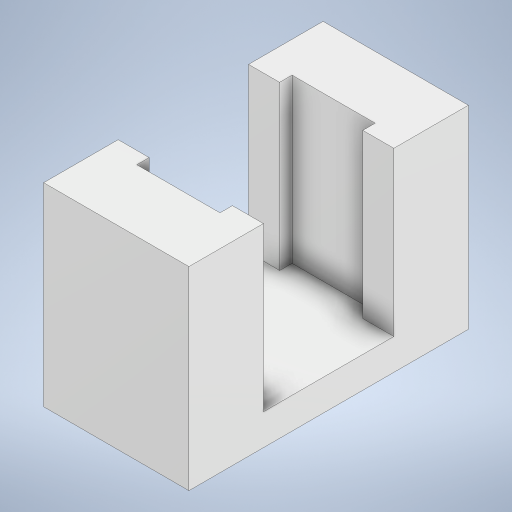
# Autodesk Inventor part: LatchSingleFit
Saved by Autodesk Inventor 2024 (Build 280153000, 153)
## iProperties
Created: 2023-10-31
Part Number: LatchSingleFit
Material: PC/ABS Plastic
Document SubType Name: Modeling
Designer: gcter
Density: 1.1 g/cm^3
Appearance: Smooth - White
Author: gcter
Autodesk Inventor part; units mm, degrees
ref_plane "YZ Plane" through (0, 0, 0) normal (1, 0, 0) x (0, 1, 0)
ref_plane "XZ Plane" through (0, 0, 0) normal (0, 1, 0) x (-1, 0, 0)
ref_plane "XY Plane" through (0, 0, 0) normal (0, 0, 1) x (1, 0, 0)
sketch "Sketch5" plane through (0, 0, 0) normal (0, 1, 0) x (-1, 0, 0)
  line L0 (0, 0) -> (-6.604, 0) construction
  line L1 (-6.604, 0) -> (-6.604, -12.7) construction
  line L2 (-6.604, -12.7) -> (0, -12.7) construction
  line L3 (0, -12.7) -> (0, 0) construction
  line L4 (2.6416, -15.24) -> (-9.2456, -15.24)
  line L5 (-9.2456, -15.24) -> (-9.2456, 2.54)
  line L6 (-9.2456, 2.54) -> (2.6416, 2.54)
  line L7 (2.6416, 2.54) -> (2.6416, -15.24)
  dimension "d22" = 6.604
  dimension "d23" = 12.7
  dimension "d24" = 2.6416
  dimension "d25" = 2.6416
  dimension "d26" = 2.54
  dimension "d27" = 2.54
  constraints: 16 end point, 4 parallel, 2 horizontal, 2 perpendicular
  measures "d22" distance between parallel lines of L1 L3
  measures "d23" distance between parallel lines of L0 L2
  measures "d24" distance between parallel lines of L5 L1
  measures "d25" distance between parallel lines of L3 L7
  measures "d26" distance between parallel lines of L6 L0
  measures "d27" distance between parallel lines of L2 L4
extrude "Extrusion3" add sketch "Sketch5" along normal blind 2.54
sketch "Sketch6" plane through (0, 2.54, 0) normal (0, 1, 0) x (1, 0, 0)
  line L0 (-2.6416, -2.54) -> (9.2456, -2.54)
  line L1 (9.2456, -2.54) -> (9.2456, 0)
  line L2 (6.7056, 0) -> (-0.1016, 0)
  line L3 (-2.6416, -0.508) -> (-2.6416, -2.54)
  line L4 (-2.6416, 15.24) -> (-2.6416, -2.54) projected
  line L5 (9.2456, -2.54) -> (9.2456, 15.24) projected
  line L6 (-2.6416, -2.54) -> (9.2456, -2.54) projected
  line L7 (-0.1016, 12.7) -> (6.7056, 12.7)
  line L8 (9.2456, 12.954) -> (9.2456, 15.24)
  line L9 (9.2456, 15.24) -> (-2.6416, 15.24)
  line L10 (-2.6416, 15.24) -> (-2.6416, 12.7)
  line L11 (9.2456, 15.24) -> (-2.6416, 15.24) projected
  line L12 (9.2456, 12.954) -> (9.2456, 11.684)
  line L13 (6.7056, 11.684) -> (6.7056, 12.7)
  line L14 (6.7056, 11.684) -> (9.2456, 11.684)
  line L15 (-2.6416, 12.7) -> (-2.6416, 11.684)
  line L16 (-2.6416, 11.684) -> (-0.1016, 11.684)
  line L17 (-0.1016, 11.684) -> (-0.1016, 12.7)
  line L18 (9.2456, 0) -> (9.2456, 1.016)
  line L19 (9.2456, 1.016) -> (6.7056, 1.016)
  line L20 (6.7056, 1.016) -> (6.7056, 0)
  line L21 (-0.1016, 0) -> (-0.1016, 1.016)
  line L22 (-0.1016, 1.016) -> (-2.6416, 1.016)
  line L23 (-2.6416, 1.016) -> (-2.6416, -0.508)
  point P0 (0, 0)
  point P1 (7.9756, 11.684)
  point P2 (9.2456, 0.508)
  point P3 (-2.6416, 15.24)
  point P4 (-2.6416, 1.016)
  point P5 (9.2456, 0)
  dimension "d30" = 2.54
  dimension "d31" = 2.54
  dimension "d32" = 2.54
  dimension "d33" = 1.016
  dimension "d35" = 2.54
  dimension "d36" = 1.016
  dimension "d37" = 1.016
  dimension "d38" = 2.54
  dimension "d39" = 2.54
  dimension "d40" = 1.016
  constraints: 40 end point, 9 collinear, 7 parallel, 4 perpendicular, 2 horizontal, 2 midpoint, 1 point on line
  measures "d30" distance between parallel lines of L2 L0
  measures "d31" distance between parallel lines of L7 L9
  measures "d32" distance between parallel lines of L5 L13
  measures "d33" distance from line of L7 point (7.976, 11.684)
  measures "d35" distance between parallel lines of L17 L4
  measures "d36" distance between parallel lines of L7 L16
  measures "d37" distance between parallel lines of L2 L19
  measures "d38" distance from line of point (9.246, 0.508) L20
  measures "d39" distance between parallel lines of L21 L23
  measures "d40" distance between parallel lines of L2 L22
extrude "Extrusion4" add sketch "Sketch6" along normal blind 13.335 contours L3 L4 L22 L21 L2 L20 L19 L5 L1 L0 | L4 L9 L5 L14 L13 L7 L17 L16
sketch "Sketch8" plane through (9.2456, 0, -15.24) normal (0, 0, -1) x (-1, 0, 0)
  line L0 (0, 0) -> (0, 15.875) projected
  line L1 (11.8872, 0) -> (0, 0) projected
  line L2 (0, 15.875) -> (11.8872, 15.875)
  line L3 (11.8872, 15.875) -> (11.8872, 0)
  line L4 (11.8872, 0) -> (0, 0)
  line L5 (0, 0) -> (0, 15.875)
  point P0 (9.2456, 0)
  constraints: 8 end point, 2 parallel, 1 horizontal, 1 perpendicular
extrude "Extrusion5" add sketch "Sketch8" along normal blind 2.54
sketch "Sketch9" plane through (-2.6416, 0, 2.54) normal (0, 0, 1) x (1, 0, 0)
  line L0 (2.54, 15.875) -> (0, 15.875) projected
  line L1 (11.8872, 0) -> (0, 0) projected
  line L2 (0, 15.875) -> (11.8872, 15.875)
  line L3 (11.8872, 15.875) -> (11.8872, 0)
  line L4 (11.8872, 0) -> (0, 0)
  line L5 (0, 0) -> (0, 15.875)
  point P0 (2.6416, 0)
  point P1 (0, 0)
  constraints: 8 end point, 2 parallel, 1 horizontal, 1 perpendicular
extrude "Extrusion6" add sketch "Sketch9" along normal blind 2.54
body "Solid3"
